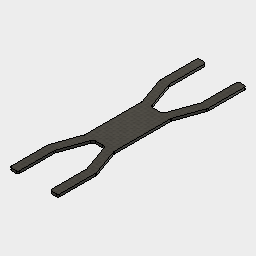
Battery Tray v2 (Autodesk Fusion 360 archive; units mm, degrees)
design "Battery Tray v2 Base"
Autodesk Fusion 360 part; units mm, degrees
sketch "Sketch1" plane through (0, 0, 0) normal (0, 1, 0) x (1, 0, 0)
  line L0 (14.8, 12) -> (14.8, -8)
  line L1 (-14.8, 12) -> (-14.8, -8)
  line L2 (-9.8, 7) -> (-9.8, -7.0489)
  line L3 (9.8, 7) -> (9.8, -7.0489)
  line L4 (9.8, 7) -> (9.8, 12)
  line L5 (-9.8, 7) -> (-9.8, 12)
  line L6 (14.8, -77.0865) -> (14.8, -97)
  line L7 (-14.8, -77.0873) -> (-14.8, -96.9944)
  line L8 (-9.8, -96.9944) -> (-9.8, -77.9519)
  line L9 (9.8, -97) -> (9.8, -77.9511)
  line L10 (4.0586, -23.6718) -> (9.6258, -8.0563)
  line L11 (-9.0092, -60.3259) -> (-14.6258, -76.0798)
  line L12 (9.0094, -60.3258) -> (14.6258, -76.079)
  line L13 (14.8, -8) -> (14.8, -7.9135)
  line L14 (14.6548, -8.8395) -> (14.6258, -8.921)
  line L15 (-14.6548, -8.8395) -> (-14.6258, -8.921)
  line L16 (-14.8, -7.9135) -> (-14.8, -8)
  line L17 (-4.0585, -23.6718) -> (-9.6258, -8.0563)
  line L18 (-9.6258, -76.9445) -> (-4.0584, -61.3286)
  line L19 (9.0094, -24.6744) -> (14.6548, -8.8395)
  line L20 (9.6258, -76.9437) -> (4.0587, -61.3286)
  line L21 (-9.0092, -24.6747) -> (-14.6548, -8.8395)
  line L22 (-9.8, 12) -> (-9.8, 14)
  line L23 (-14.8, 14) -> (-14.8, 12)
  line L24 (14.8, 12) -> (14.8, 14)
  line L25 (9.8, 14) -> (9.8, 12)
  line L26 (-9.8, -96.9944) -> (-9.8, -98.9944)
  line L27 (-14.8, -98.9944) -> (-14.8, -96.9944)
  line L28 (14.8, -97) -> (14.8, -99)
  line L29 (9.8, -99) -> (9.8, -97)
  line L30 (2.1747, -25.0002) -> (-2.1747, -25.0002)
  line L31 (-8.8931, -25.3464) -> (-8.8931, -59.6542)
  line L32 (-2.1746, -60.0002) -> (2.1748, -60.0002)
  line L33 (8.8933, -59.6541) -> (8.8933, -25.3461)
  arc A0 (-8.8931, -25.3464) -> (-9.0092, -24.6747) centre (-10.8931, -25.3464) ccw
  arc A1 (-4.0585, -23.6718) -> (-2.1747, -25.0002) centre (-2.1747, -23.0002) ccw
  arc A2 (2.1747, -25.0002) -> (4.0586, -23.6718) centre (2.1747, -23.0002) ccw
  arc A3 (9.0094, -24.6744) -> (8.8933, -25.3461) centre (10.8933, -25.3461) ccw
  arc A4 (8.8933, -59.6541) -> (9.0094, -60.3258) centre (10.8933, -59.6541) ccw
  arc A5 (4.0587, -61.3286) -> (2.1748, -60.0002) centre (2.1748, -62.0002) ccw
  arc A6 (-2.1746, -60.0002) -> (-4.0584, -61.3286) centre (-2.1746, -62.0002) ccw
  arc A7 (-9.0092, -60.3259) -> (-8.8931, -59.6542) centre (-10.8931, -59.6542) ccw
  arc A8 (-14.6258, -76.0798) -> (-14.8, -77.0873) centre (-11.8, -77.0873) ccw
  arc A9 (-9.6258, -76.9445) -> (-9.8, -77.9519) centre (-6.8, -77.9519) ccw
  arc A10 (9.8, -77.9511) -> (9.6258, -76.9437) centre (6.8, -77.9511) ccw
  arc A11 (14.8, -77.0865) -> (14.6258, -76.079) centre (11.8, -77.0865) ccw
  arc A12 (14.6258, -8.921) -> (14.8, -7.9135) centre (11.8, -7.9135) ccw
  arc A13 (9.6258, -8.0563) -> (9.8, -7.0489) centre (6.8, -7.0489) ccw
  arc A14 (-9.8, -7.0489) -> (-9.6258, -8.0563) centre (-6.8, -7.0489) ccw
  arc A15 (-14.8, -7.9135) -> (-14.6258, -8.921) centre (-11.8, -7.9135) ccw
  line L34 (-10.8, 15) -> (-13.8, 15)
  line L35 (10.8, 15) -> (13.8, 15)
  line L36 (10.8, -100) -> (13.8, -100)
  line L37 (-10.8, -99.9944) -> (-13.8, -99.9944)
  arc A16 (-14.8, -98.9944) -> (-13.8, -99.9944) centre (-13.8, -98.9944) ccw
  arc A17 (-10.8, -99.9944) -> (-9.8, -98.9944) centre (-10.8, -98.9944) ccw
  arc A18 (9.8, -99) -> (10.8, -100) centre (10.8, -99) ccw
  arc A19 (13.8, -100) -> (14.8, -99) centre (13.8, -99) ccw
  arc A20 (14.8, 14) -> (13.8, 15) centre (13.8, 14) ccw
  arc A21 (-13.8, 15) -> (-14.8, 14) centre (-13.8, 14) ccw
  arc A22 (10.8, 15) -> (9.8, 14) centre (10.8, 14) ccw
  arc A23 (-9.8, 14) -> (-10.8, 15) centre (-10.8, 14) ccw
  point P0 (0.0001, -42.5002)
  dimension "d39" = 1
  measures "d39" radius of A16
extrude "Extrude1" add sketch "Sketch1" along normal blind 1.5

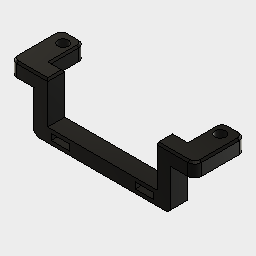
design "Battery Tray v2 Back"
Autodesk Fusion 360 part; units mm, degrees
sketch "Sketch1" plane through (0, 0, 0) normal (0, 1, 0) x (1, 0, 0)
  line L0 (-27, 17) -> (-27, 14)
  line L1 (-27, 17) -> (-27, 25)
  line L2 (-25, 27) -> (-22, 27)
  circle A0 centre (-23, 23.5) radius 1.55
  line L3 (-20, 25) -> (-20, 17)
  line L4 (-25, 12) -> (-20, 12)
  line L5 (20, 12) -> (-20, 12)
  line L6 (-20, 17) -> (20, 17)
  line L7 (25, 12) -> (20, 12)
  line L8 (27, 17) -> (27, 14)
  line L9 (27, 17) -> (27, 25)
  line L10 (20, 25) -> (20, 17)
  line L11 (25, 27) -> (22, 27)
  circle A1 centre (23, 23.5) radius 1.55
  line L12 (-20, 17) -> (-20, 12)
  line L13 (20, 17) -> (20, 12)
  line L14 (-20, 17) -> (-16, 17)
  line L15 (-16, 17) -> (-16, 12)
  line L16 (-16, 12) -> (-20, 12)
  line L17 (-20, 12) -> (-20, 17)
  line L18 (20, 17) -> (16, 17)
  line L19 (16, 17) -> (16, 12)
  line L20 (16, 12) -> (20, 12)
  line L21 (20, 12) -> (20, 17)
  arc A2 (-25, 27) -> (-27, 25) centre (-25, 25) ccw
  arc A3 (-20, 25) -> (-22, 27) centre (-22, 25) ccw
  arc A4 (-27, 14) -> (-25, 12) centre (-25, 14) ccw
  arc A5 (25, 12) -> (27, 14) centre (25, 14) ccw
  arc A6 (27, 25) -> (25, 27) centre (25, 25) ccw
  arc A7 (22, 27) -> (20, 25) centre (22, 25) ccw
  dimension "d1" = 5
  dimension "d4" = 4
  dimension "d5" = 5
  dimension "d6" = 4
  dimension "d9" = 2
  measures "d1" distance of L3.end L4.end
  measures "d4" distance of L3.end L14.end
  measures "d5" distance of L3.end L4.end
  measures "d6" distance of L6.end L18.end
  measures "d9" radius of A2
extrude "Extrude3" add sketch "Sketch1" along normal blind 4 contours L0 L1 L2 L3 L4 L12 L17 A2 A3 A4 | L5 L6 L12 L14 L15 L16 L17 | L5 L6 L13 L18 L19 L20 L21 | L7 L8 L9 L10 L11 L13 L21 A5 A6 A7 makes body 1 at (-23.3719, 0, -18.6514) makes body 2 at (23.3719, 0, -18.6514)
extrude "Extrude4" add sketch "Sketch1" against normal blind 8 contours L5 L6 L12 L14 L15 L16 L17 | L5 L6 L13 L18 L19 L20 L21 bodies 1 2
sketch "Sketch2" plane through (0, -8, 0) normal (0, -1, 0) x (1, 0, 0)
  line L0 (-16, -12) -> (-20, -12)
  line L1 (-20, -12) -> (-20, -17)
  line L2 (-20, -17) -> (-16, -17)
  line L3 (-16, -17) -> (-16, -12)
  line L4 (-20, -12) -> (20, -12)
  line L5 (20, -12) -> (20, -17)
  line L6 (20, -17) -> (-20, -17)
  line L7 (-20, -17) -> (-20, -12)
  point P0 (20, -17)
extrude "Extrude5" add sketch "Sketch2" along normal blind 4 bodies 1 2
sketch "Sketch3" plane through (0, 0, -12) normal (0, 0, 1) x (1, 0, 0)
  line L0 (-25, 0) -> (-20, 0)
  line L1 (-20, 0) -> (-20, -12)
  line L2 (-20, -12) -> (20, -12)
  line L3 (20, -12) -> (20, 0)
  line L4 (20, 0) -> (25, 0)
  line L5 (25, 0) -> (25, 4)
  line L6 (25, 4) -> (16, 4)
  line L7 (16, 4) -> (16, -8)
  line L8 (16, -8) -> (-16, -8)
  line L9 (-16, -8) -> (-16, 4)
  line L10 (-16, 4) -> (-25, 4)
  line L11 (-25, 4) -> (-25, 0)
  line L12 (9.6, -9.1) -> (15, -9.1)
  line L13 (-9.6, -9.1) -> (-9.6, -10.9)
  line L14 (15, -10.9) -> (9.6, -10.9)
  line L15 (9.6, -10.9) -> (9.6, -9.1)
  line L16 (-15, -9.1) -> (-9.6, -9.1)
  line L17 (-9.6, -10.9) -> (-15, -10.9)
  line L18 (-15, -10.9) -> (-15, -9.1)
  line L19 (15, -9.1) -> (15, -10.9)
  dimension "d16" = 5.4
  dimension "d17" = 1.8
  dimension "d18" = 5.4
  dimension "d19" = 1.8
  dimension "d20" = 5
  dimension "d21" = 5
  dimension "d22" = 1.1
  dimension "d23" = 1.1
  measures "d16" distance of L14.start L14.end
  measures "d17" distance of L14.start L12.end
  measures "d18" distance of L13.end L17.end
  measures "d19" distance of L13.end L13.start
  measures "d20" distance of L3 L19
  measures "d21" distance of L1 L18
  measures "d22" distance of L8 L16
  measures "d23" distance of L8 L12
extrude "Extrude6" cut sketch "Sketch3" against normal blind 4 contours L12 L14 L15 L19 | L13 L16 L17 L18 bodies 1
chamfer "Chamfer1" distance 1 angle 45 2 edges at (-20, -12, -14.5) (20, -12, -14.5) on bodies 1
chamfer "Chamfer2" distance 0.5 angle 45 18 edges at (-16, 4, -14.5) (-20, 4, -21) (-20.5858, 4, -26.4142) (-23.5, 4, -27) (-26.4142, 4, -26.4142) (-27, 4, -19.5) (-26.4142, 4, -12.5858) (-20.5, 4, -12) (-18, 4, -17) (20.5, 4, -12) (26.4142, 4, -12.5858) (27, 4, -19.5) (26.4142, 4, -26.4142) (23.5, 4, -27) (20.5858, 4, -26.4142) (20, 4, -21) (18, 4, -17) (16, -2, -17) on bodies 1 2

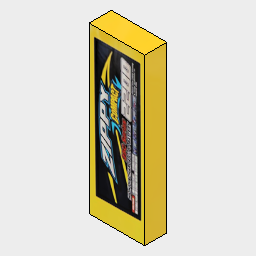
design "Battery"
Autodesk Fusion 360 part; units mm, degrees
sketch "Sketch1" plane through (0, 0, 0) normal (0, 1, 0) x (1, 0, 0)
  line L0 (0, 0) -> (35, 0)
  line L1 (35, 0) -> (35, -14)
  line L2 (0, -14) -> (0, 0)
  line L3 (0, 0) -> (35, 0)
  line L4 (35, 0) -> (35, -14)
  line L5 (35, -14) -> (0, -14)
  line L6 (0, -14) -> (0, 0)
  dimension "d6" = 35
  dimension "d8" = 14
  measures "d6" distance of L0.start L0.end
  measures "d8" distance of L0.start L2.start
extrude "Extrude1" add sketch "Sketch1" along normal blind 104
